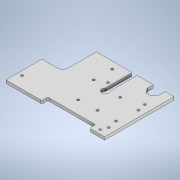
# Autodesk Inventor part: Bottle side plate
Saved by Autodesk Inventor 2021 (Build 250183000, 183)
## iProperties
Created: 2020-08-12
Part Number: Bottle side plate
Material: Generic
Document SubType Name: Modeling
Designer: jgray
Density: 1 g/cm^3
Appearance: Default
Author: jgray
Autodesk Inventor part; units mm, degrees
ref_plane "YZ Plane" through (0, 0, 0) normal (1, 0, 0) x (0, 1, 0)
ref_plane "XZ Plane" through (0, 0, 0) normal (0, 1, 0) x (-1, 0, 0)
ref_plane "XY Plane" through (0, 0, 0) normal (0, 0, 1) x (1, 0, 0)
sketch "Sketch1" plane through (0, 0, 0) normal (0, 1, 0) x (-1, 0, 0)
  line L0 (0, 0) -> (130, 0)
  line L1 (130, 0) -> (130, -116.2)
  line L2 (130, -116.2) -> (0, -116.2)
  line L3 (0, -116.2) -> (0, 0)
  dimension "d0" = 130
  dimension "d1" = 116.2
  constraints: 8 end point, 2 parallel, 1 horizontal, 1 perpendicular
  measures "d0" distance of L1.end L2.end
  measures "d1" distance of L0.end L1.end
extrude "Extrusion1" add sketch "Sketch1" along normal blind 5
sketch "Sketch2" plane through (0, 5, 0) normal (0, 1, 0) x (1, 0, 0)
  line L0 (-10, -25.3077) -> (-10, 177.8334) construction
  line L1 (0, 0) -> (0, 116.2) construction
  line L2 (-130, 0) -> (0, 0) construction
  line L3 (-47, -19.5328) -> (-47, 162.8865) construction
  line L4 (0, 116.2) -> (-130, 116.2) construction
  point P0 (-10, 16.7)
  point P1 (-10, 66.7)
  point P2 (-47, 111.7)
  point P3 (-47, 43.95)
  point P4 (-47, 17.95)
  dimension "d4" = 10
  dimension "d5" = 16.7
  dimension "d6" = 50
  dimension "d7" = 47
  dimension "d8" = 4.5
  dimension "d9" = 72.25
  dimension "d10" = 98.25
  constraints: 5 point on line, 4 end point, 2 vertical
  measures "d4" distance between parallel lines of L1 L0
  measures "d5" distance from line of L2 point (-10, 16.7)
  measures "d6" distance of point (-10, 66.7) point (-10, 16.7)
  measures "d7" distance between parallel lines of L3 L1
  measures "d8" distance from line of L4 point (-47, 111.7)
  measures "d9" distance from line of point (-47, 43.95) L4
  measures "d10" distance from line of point (-47, 17.95) L4
hole "Hole1" at (-10, 5, -16.7) at (-10, 5, -66.7) direction (0, -1, 0) diameter 3.8 end through all
sketch "Sketch3" plane through (0, 5, 0) normal (0, 1, 0) x (1, 0, 0)
  line L0 (-105, 0) -> (-25, 0)
  line L1 (-25, 0) -> (-25, 8)
  line L2 (-27, 10) -> (-103, 10)
  line L3 (-105, 8) -> (-105, 0)
  line L4 (-130, 116.2) -> (-130, 0) projected
  line L5 (0, 0) -> (0, 116.2) projected
  arc A0 (-103, 10) -> (-105, 8) centre (-103, 8) ccw
  arc A1 (-25, 8) -> (-27, 10) centre (-27, 8) ccw
  dimension "d18" = 10
  dimension "d19" = 25
  dimension "d20" = 25
  dimension "d21" = 2
  constraints: 8 end point, 4 point on circle, 4 tangent, 2 centre point, 2 parallel, 1 equal radius, 1 horizontal, 1 perpendicular
  measures "d18" distance between parallel lines of L0 L2
  measures "d19" distance between parallel lines of L4 L3
  measures "d20" distance between parallel lines of L5 L1
  measures "d21" radius of A0
extrude "Extrusion2" cut sketch "Sketch3" against normal blind 5
fillet "Fillet1" radius 2 2 edges at (-105, 2.5, 0) (-25, 2.5, 0)
sketch "Sketch4" plane through (0, 5, 0) normal (0, 1, 0) x (1, 0, 0)
  circle A0 centre (-65.75, 67.1) radius 6
  line L0 (0, 0) -> (0, 116.2) projected
  line L1 (-23, 0) -> (0, 0) projected
  dimension "d25" = 12
  dimension "d26" = 65.75
  dimension "d27" = 67.1
  constraints: 1 centre point
  measures "d25" diameter of A0
  measures "d26" distance from line of L0 A0.centre
  measures "d27" distance from line of L1 A0.centre
extrude "Extrusion3" cut sketch "Sketch4" against normal blind 5
sketch "Sketch5" plane through (0, 5, 0) normal (0, 1, 0) x (1, 0, 0)
  line L0 (-91.5, 130.6682) -> (-91.5, -27.2079) construction
  line L1 (0, 0) -> (0, 116.2) construction
  line L2 (0, 116.2) -> (-130, 116.2) construction
  point P0 (-91.5, 104.2)
  point P1 (-91.5, 73.2)
  dimension "d30" = 91.5
  dimension "d31" = 12
  dimension "d32" = 43
  constraints: 2 end point, 2 point on line, 1 vertical
  measures "d30" distance between parallel lines of L1 L0
  measures "d31" distance from line of L2 point (-91.5, 104.2)
  measures "d32" vertical distance of L2.end point (-91.5, 73.2)
hole "Hole2" at (-91.5, 5, -104.2) at (-91.5, 5, -73.2) direction (0, -1, 0) diameter 3.8 end through all
sketch "Sketch6" plane through (0, 5, 0) normal (0, 1, 0) x (1, 0, 0)
  line L0 (-13, 148.9997) -> (-13, -38.8385) construction
  line L1 (0, 0) -> (0, 116.2) projected
  line L2 (0, 116.2) -> (-130, 116.2) projected
  line L3 (-44, 144.1508) -> (-44, -38.8385) construction
  line L4 (-14, 12.9628) -> (-14, -11.5017) construction
  line L5 (-23, 0) -> (0, 0) construction
  point P0 (-13, 80.2)
  point P1 (-13, 32.2)
  point P2 (-44, 70.2)
  point P3 (-44, 32.2)
  point P4 (-14, 6.7)
  dimension "d40" = 13
  dimension "d41" = 36
  dimension "d42" = 84
  dimension "d50" = 44
  dimension "d51" = 46
  dimension "d52" = 84
  dimension "d53" = 14
  dimension "d54" = 6.7
  constraints: 6 end point, 5 point on line, 3 vertical
  measures "d40" distance between parallel lines of L1 L0
  measures "d41" distance from line of point (-13, 80.2) L2
  measures "d42" distance from line of L2 point (-13, 32.2)
  measures "d50" distance between parallel lines of L1 L3
  measures "d51" distance from line of L2 point (-44, 70.2)
  measures "d52" distance from line of point (-44, 32.2) L2
  measures "d53" distance between parallel lines of L1 L4
  measures "d54" distance from line of L5 point (-14, 6.7)
hole "Hole3" at (-13, 5, -80.2) at (-13, 5, -32.2) at (-44, 5, -32.2) at (-44, 5, -70.2) at (-14, 5, -6.7) direction (0, -1, 0) diameter 3.8 end through all
sketch "Sketch7" plane through (-130, 0, -116.2) normal (-1, 0, 0) x (0, 0, 1)
  line L0 (116.2, 0) -> (56.2, 0)
  line L1 (56.2, 0) -> (56.2, 5)
  line L2 (56.2, 5) -> (116.2, 5)
  line L3 (116.2, 5) -> (116.2, 0)
  dimension "d55" = 60
  dimension "d56" = 5
  constraints: 8 end point, 2 parallel, 1 horizontal, 1 perpendicular
  measures "d55" distance of L1.end L2.end
  measures "d56" distance of L0.end L1.end
extrude "Extrusion4" add sketch "Sketch7" along normal blind 35
fillet "Fillet2" radius 10 1 edges at (-130, 2.5, -60)
sketch "Sketch8" plane through (0, 5, 0) normal (0, 1, 0) x (1, 0, 0)
  line L0 (-107, 0) -> (-165, 0) projected
  line L1 (-165, 0) -> (-165, 60) projected
  point P0 (0, 0)
  point P1 (-157.75, 19.5)
  dimension "d60" = 19.5
  dimension "d61" = 7.25
  measures "d60" distance from line of L0 point (-157.75, 19.5)
  measures "d61" distance from line of L1 point (-157.75, 19.5)
hole "Hole4" at (-157.75, 5, -19.5) direction (0, -1, 0) diameter 3.8 end through all
sketch "Sketch9" plane through (0, 5, 0) normal (0, 1, 0) x (1, 0, 0)
  line L0 (-24.65, 135.1246) -> (-24.65, 98.3323) construction
  line L1 (0, 0) -> (0, 116.2) projected
  line L2 (-34.65, 134.2) -> (-14.65, 134.2)
  line L3 (-14.65, 134.2) -> (-14.65, 98.2)
  line L4 (-14.65, 98.2) -> (-34.65, 98.2)
  line L5 (-34.65, 98.2) -> (-34.65, 134.2)
  line L6 (0, 116.2) -> (-130, 116.2) projected
  line L7 (-34.65, 134.2) -> (-14.65, 98.2) construction
  line L8 (-14.65, 134.2) -> (-34.65, 98.2) construction
  line L9 (-14.65, 106.2) -> (-20.65, 98.2)
  line L10 (-34.65, 106.2) -> (-28.65, 98.2)
  line L11 (-34.65, 116.2) -> (-14.65, 116.2)
  point P0 (-24.65, 116.2)
  dimension "d69" = 24.65
  dimension "d70" = 20
  dimension "d71" = 36
  dimension "d72" = 10
  dimension "d73" = 8
  constraints: 20 end point, 8 point on line, 4 midpoint, 2 parallel, 1 horizontal, 1 perpendicular, 1 vertical, 1 other
  measures "d69" distance between parallel lines of L1 L0
  measures "d70" distance of L3.end L4.end
  measures "d71" distance of L2.end L3.end
  measures "d72" distance from line of L6 L9.start
  measures "d73" distance of L9.end L10.end
extrude "Extrusion5" cut sketch "Sketch9" against normal through all contours L6 L3 L9 L4 L10 L5
fillet "Fillet3" radius 2 4 edges at (-34.65, 2.5, -106.2) (-28.65, 2.5, -98.2) (-20.65, 2.5, -98.2) (-14.65, 2.5, -106.2)
sketch "Sketch10" plane through (0, 5, 0) normal (0, 1, 0) x (1, 0, 0)
  line L0 (-34.65, 106.8667) -> (-34.65, 116.2) projected
  line L1 (-34.65, 116.2) -> (-130, 116.2) projected
  line L2 (-130, 116.2) -> (-130, 70) projected
  arc A0 (-140, 60) -> (-130, 70) centre (-140, 70) ccw projected
  line L3 (-140, 60) -> (-165, 60) projected
  line L4 (-165, 0) -> (-165, 60) projected
  line L5 (-107, 0) -> (-165, 0) projected
  arc A1 (-107, 0) -> (-105, 2) centre (-107, 2) ccw projected
  line L6 (-105, 2) -> (-105, 8) projected
  arc A2 (-103, 10) -> (-105, 8) centre (-103, 8) ccw projected
  line L7 (-103, 10) -> (-27, 10) projected
  arc A3 (-25, 8) -> (-27, 10) centre (-27, 8) ccw projected
  line L8 (-25, 8) -> (-25, 2) projected
  arc A4 (-25, 2) -> (-23, 0) centre (-23, 2) ccw projected
  line L9 (-23, 0) -> (0, 0) projected
  line L10 (0, 0) -> (0, 116.2) projected
  line L11 (0, 116.2) -> (-14.65, 116.2) projected
  line L12 (-14.65, 116.2) -> (-14.65, 106.8667) projected
  arc A5 (-15.05, 105.6667) -> (-14.65, 106.8667) centre (-16.65, 106.8667) ccw projected
  line L13 (-15.05, 105.6667) -> (-20.05, 99) projected
  arc A6 (-21.65, 98.2) -> (-20.05, 99) centre (-21.65, 100.2) ccw projected
  line L14 (-21.65, 98.2) -> (-27.65, 98.2) projected
  arc A7 (-29.25, 99) -> (-27.65, 98.2) centre (-27.65, 100.2) ccw projected
  line L15 (-29.25, 99) -> (-34.25, 105.6667) projected
  arc A8 (-34.65, 106.8667) -> (-34.25, 105.6667) centre (-32.65, 106.8667) ccw projected
  circle A9 centre (-157.75, 19.5) radius 1.9 projected
  circle A10 centre (-44, 70.2) radius 1.9 projected
  circle A11 centre (-13, 32.2) radius 1.9 projected
  circle A12 centre (-13, 80.2) radius 1.9 projected
  circle A13 centre (-44, 32.2) radius 1.9 projected
  circle A14 centre (-14, 6.7) radius 1.9 projected
  circle A15 centre (-91.5, 104.2) radius 1.9 projected
  circle A16 centre (-91.5, 73.2) radius 1.9 projected
  circle A17 centre (-65.75, 67.1) radius 6 projected
  circle A18 centre (-10, 16.7) radius 1.9 projected
  circle A19 centre (-10, 66.7) radius 1.9 projected
  line L16 (-65.75, 187.4389) -> (-65.75, -19.4667) construction
  line L17 (-34.65, 116.2) -> (-130, 116.2) projected
  circle A20 centre (-65.75, 67.1) radius 6 projected
  line L18 (-69.75, 116.2) -> (-61.75, 116.2)
  line L19 (-61.75, 116.2) -> (-61.75, 71.5721)
  line L20 (-61.75, 71.5721) -> (-69.75, 71.5721)
  line L21 (-69.75, 71.5721) -> (-69.75, 116.2)
  dimension "d77" = 8
  constraints: 10 end point, 2 parallel, 2 point on line, 1 horizontal, 1 perpendicular, 1 vertical, 5 other
  measures "d77" distance between parallel lines of L19 L21
extrude "Extrusion6" cut sketch "Sketch10" against normal through all contours L19 A17 L21 L1
fillet "Fillet4" radius 2 4 edges at (-69.75, 2.5, -116.2) (-61.75, 2.5, -116.2) (-69.75, 2.5, -71.5721) (-61.75, 2.5, -71.5721)
sketch "Sketch11" plane through (0, 5, 0) normal (0, 1, 0) x (1, 0, 0)
  line L0 (-75.5, 139.1066) -> (-75.5, -104.8745) construction
  line L1 (0, 0) -> (0, 116.2) construction
  line L2 (-71.75, 116.2) -> (-130, 116.2) construction
  point P0 (-75.5, 31.2)
  point P1 (-75.5, 81.2)
  dimension "d81" = 75.5
  dimension "d82" = 35
  dimension "d83" = 85
  constraints: 2 end point, 2 point on line, 1 vertical
  measures "d81" distance between parallel lines of L0 L1
  measures "d82" distance from line of point (-75.5, 81.2) L2
  measures "d83" distance from line of point (-75.5, 31.2) L2
hole "Hole5" at (-75.5, 5, -31.2) at (-75.5, 5, -81.2) direction (0, -1, 0) diameter 3.8 end through all
body "Solid1"
